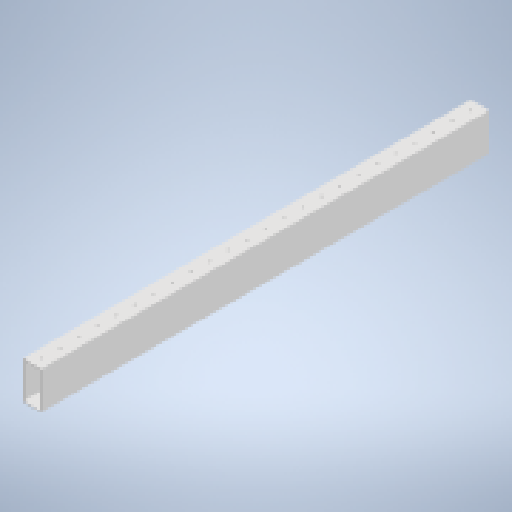
# Autodesk Inventor part: Long bar 3- VersaFrame
Saved by Autodesk Inventor 2024 (Build 280153000, 153)
## iProperties
Created: 2020-01-13
Part Number: Long bar 3- VersaFrame
Material: Generic
Document SubType Name: Modeling
Designer: aidan
Density: 1 g/cm^3
Appearance: Default
Author: aidan
Autodesk Inventor part; units mm, degrees
ref_plane "YZ Plane" through (0, 0, 0) normal (1, 0, 0) x (0, 1, 0)
ref_plane "XZ Plane" through (0, 0, 0) normal (0, 1, 0) x (-1, 0, 0)
ref_plane "XY Plane" through (0, 0, 0) normal (0, 0, 1) x (1, 0, 0)
sketch "Sketch1" plane through (0, 0, 0) normal (0, 0, 1) x (1, 0, 0)
  line L0 (-12.1708, 16.0073) -> (13.2292, 16.0073)
  line L1 (13.2292, 16.0073) -> (13.2292, -34.7927)
  line L2 (13.2292, -34.7927) -> (-12.1708, -34.7927)
  line L3 (-12.1708, -34.7927) -> (-12.1708, 16.0073)
  line L4 (11.9592, 14.7373) -> (-10.9008, 14.7373)
  line L5 (-10.9008, 14.7373) -> (-10.9008, -33.5227)
  line L6 (-10.9008, -33.5227) -> (11.9592, -33.5227)
  line L7 (11.9592, -33.5227) -> (11.9592, 14.7373)
  point P0 (0, 0)
  dimension "d0" = 25.4
  dimension "d1" = 50.8
  dimension "d2" = 1.27
  constraints: 16 end point, 4 parallel, 2 perpendicular, 1 horizontal, 3 other
  measures "d0" distance of L0.start L0.end
  measures "d1" distance of L0.end L1.end
  measures "d2" distance between parallel lines of L0 L4
extrude "Extrusion1" add sketch "Sketch1" along normal blind 609.6
sketch "Sketch2" plane through (-12.1708, 16.0073, 0) normal (0, 1, 0) x (1, 0, 0)
  circle A0 centre (12.7, -12.7) radius 1.7272
  line L0 (25.4, 0) -> (0, 0) projected
  line L1 (0, 0) -> (0, -609.6) projected
  point P0 (12.1708, 0)
  dimension "d5" = 3.4544
  dimension "d6" = 12.7
  dimension "d7" = 12.7
  constraints: 1 centre point
  measures "d5" diameter of A0
  measures "d6" distance from line of L0 A0.centre
  measures "d7" distance from line of L1 A0.centre
extrude "Extrusion2" cut sketch "Sketch2" against normal through all
pattern_linear "Rectangular Pattern1" count 61 spacing 25.4 along (0, 0, 1) of "Extrusion2"
sketch "Sketch6" plane through (-12.1708, -34.7927, 0) normal (-1, 0, 0) x (0, 0, 1)
  circle A0 centre (203.2, 25.4) radius 2.3813
  circle A1 centre (177.8, 25.4) radius 2.3813
  circle A2 centre (152.4, 25.4) radius 2.3813
  line L0 (152.4, 25.4) -> (203.2, 25.4)
  line L1 (0, 50.8) -> (0, 0) projected
  line L2 (0, 50.8) -> (609.6, 50.8) projected
  circle A3 centre (596.9, 25.4) radius 2.3813
  circle A4 centre (584.2, 25.4) radius 2.3813
  circle A5 centre (571.5, 25.4) radius 2.3813
  line L3 (571.5, 25.4) -> (596.9, 25.4)
  line L4 (609.6, 50.8) -> (609.6, 0) projected
  point P0 (0, 34.7927)
  dimension "d38" = 4.7625
  dimension "d39" = 50.8
  dimension "d41" = 25.4
  dimension "d43" = 152.4
  dimension "d44" = 4.7625
  dimension "d45" = 25.4
  dimension "d46" = 25.4
  dimension "d47" = 12.7
  constraints: 6 centre point, 6 coincident, 4 end point, 4 equal radius, 2 horizontal, 2 midpoint
  measures "d38" diameter of A1
  measures "d39" distance of L0.start L0.end
  measures "d41" distance from line of L2 A1.centre
  measures "d43" distance from line of L1 A2.centre
  measures "d44" diameter of A4
  measures "d45" distance of L3.start L3.end
  measures "d46" distance from line of A4.centre L2
  measures "d47" distance from line of L4 A3.centre
extrude "Extrusion6" cut sketch "Sketch6" against normal through all
sketch "Sketch7" plane through (-12.1708, -34.7927, 0) normal (-1, 0, 0) x (0, 0, 1)
  circle A0 centre (63.5, 25.4) radius 14.2875
  line L0 (0, 50.8) -> (0, 0) projected
  line L1 (0, 0) -> (609.6, 0) projected
  point P0 (0, 34.7927)
  dimension "d50" = 63.5
  dimension "d51" = 25.4
  dimension "d52" = 28.575
  constraints: 1 centre point
  measures "d50" distance from line of L0 A0.centre
  measures "d51" distance from line of L1 A0.centre
  measures "d52" diameter of A0
extrude "Extrusion7" cut sketch "Sketch7" against normal through all
equation "\"d3\" = d13"
equation "\"d10\" = d14"
equation "\"d13\" = 609.6"
equation "\"d14\" = d13"
body "Solid1"
